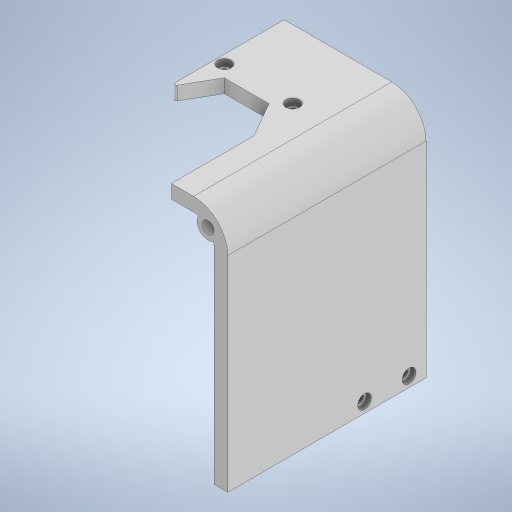
# Autodesk Inventor part: 배터리 커버
Saved by Autodesk Inventor 2023 (Build 270158000, 158)
## iProperties
Created: 2022-08-16
Part Number: 배터리 커버
Material: 일반
Document SubType Name: Modeling
Designer: fly01
Density: 1 g/cm^3
Appearance: 기본값
Author: fly01
Autodesk Inventor part; units mm, degrees
ref_plane "YZ Plane" through (0, 0, 0) normal (1, 0, 0) x (0, 1, 0)
ref_plane "XZ Plane" through (0, 0, 0) normal (0, 1, 0) x (-1, 0, 0)
ref_plane "XY Plane" through (0, 0, 0) normal (0, 0, 1) x (1, 0, 0)
sketch "스케치1" plane through (0, 0, 0) normal (0, 0, 1) x (1, 0, 0)
  line L0 (-7.2322, -10.1) -> (-7.2322, -70.1)
  line L1 (-17.2322, -0.1) -> (-48.7322, -0.1)
  line L2 (-34.3093, -4.1) -> (-17.2322, -4.1)
  line L3 (-11.2322, -10.1) -> (-11.2322, -70.1)
  line L4 (-48.7322, -0.1) -> (-48.7322, -4.1)
  line L5 (-48.7322, -4.1) -> (-34.3093, -4.1)
  line L6 (-11.2322, -70.1) -> (-7.2322, -70.1)
  arc A0 (-11.2322, -10.1) -> (-17.2322, -4.1) centre (-17.2322, -10.1) ccw
  arc A1 (-7.2322, -10.1) -> (-17.2322, -0.1) centre (-17.2322, -10.1) ccw
  point P0 (-7.2322, -0.1)
  dimension "d0" = 70
  dimension "d1" = 41.5
  dimension "d2" = 4
  dimension "d3" = 90
  dimension "d4" = 6
  dimension "d5" = 10
  constraints: 14 end point, 4 point on circle, 4 tangent, 3 horizontal, 2 centre point, 2 point on line, 1 vertical, 1 other
  measures "d0" distance of point (-7.232, -0.1) L0.end
  measures "d1" distance of point (-7.232, -0.1) L1.end
  measures "d2" distance between parallel lines of L1 L2
  measures "d3" angle of L4 L5
  measures "d4" radius of A0
  measures "d5" radius of A1
extrude "돌출1" add sketch "스케치1" along normal blind 23
sketch "스케치2" plane through (-7.2322, -70.1, 0) normal (1, 0, 0) x (0, 0, -1)
  line L0 (-23, 0) -> (-23, 60) projected
  line L1 (-23, 6) -> (0, 6)
  line L2 (0, 60) -> (0, 0) projected
  line L3 (0, 6) -> (0, 0)
  line L4 (0, 3) -> (-23, 3) construction
  line L5 (0, 0) -> (-23, 0) projected
  circle A0 centre (-18, 3) radius 1.25
  circle A1 centre (-5, 3) radius 1.25
  point P0 (0, 70.1)
  dimension "d8" = 6
  dimension "d9" = 2.5
  dimension "d10" = 2.5
  dimension "d11" = 5
  dimension "d12" = 5
  constraints: 6 end point, 4 point on line, 2 centre point, 2 perpendicular, 1 horizontal, 1 midpoint
  measures "d8" distance between parallel lines of L5 L1
  measures "d9" diameter of A0
  measures "d10" diameter of A1
  measures "d11" distance from line of L0 A0.centre
  measures "d12" distance from line of L2 A1.centre
extrude "돌출2" cut sketch "스케치2" against normal through all contours A0 | A1
sketch "스케치3" plane through (-7.2322, -70.1, 0) normal (1, 0, 0) x (0, 0, -1)
  circle A0 centre (-18, 3) radius 1.25 projected
  circle A1 centre (-18, 3) radius 2
  circle A2 centre (-5, 3) radius 1.25 projected
  circle A3 centre (-5, 3) radius 2
  point P0 (0, 70.1)
  dimension "d15" = 4
  dimension "d16" = 4
  constraints: 2 centre point, 2 coincident
  measures "d15" diameter of A1
  measures "d16" diameter of A3
extrude "돌출3" cut sketch "스케치3" against normal blind 1.5 contours A0 | A1 | A2 | A3
sketch "스케치4" plane through (-48.7322, -0.1, 0) normal (0, 1, 0) x (1, 0, 0)
  line L0 (0, -34.8253) -> (6.25, -24)
  line L1 (6.25, -24) -> (18.75, -24)
  line L2 (18.75, -24) -> (25, -34.8253)
  line L3 (25, -34.8253) -> (18.75, -45.6506)
  line L4 (18.75, -45.6506) -> (6.25, -45.6506)
  line L5 (6.25, -45.6506) -> (0, -34.8253)
  line L6 (0, 0) -> (0, -23) projected
  line L7 (0, -34.8253) -> (0, -23)
  line L8 (25, -34.8253) -> (25, -17.3222)
  line L9 (0, -23) -> (31.5, -23) projected
  line L10 (25.433, -34.5753) -> (19.0387, -23.5)
  line L11 (19.0387, -23.5) -> (5.9613, -23.5)
  line L12 (5.9613, -23.5) -> (-0.433, -34.5753)
  point P0 (48.7322, 0)
  point P1 (12.5, -34.8253)
  point P2 (15.75, -23)
  point P3 (25, -23)
  point P4 (25, -33.8253)
  point P5 (0, -33.8253)
  dimension "d19" = 25
  dimension "d20" = 1
  dimension "d23" = 0.5
  constraints: 22 end point, 2 vertical, 1 horizontal, 1 vertical alignment, 17 other
  measures "d19" distance of L2.end L0.start
  measures "d20" distance from line of point (15.75, -23) L1
  measures "d23" distance between parallel lines of L2 L10
extrude "돌출4" add sketch "스케치4" against normal blind 4 contours L7 L9 L8 L10 L11 L12
sketch "스케치5" plane through (0, 0, 23) normal (0, 0, 1) x (1, 0, 0)
  line L0 (-23.7322, -0.1) -> (-23.7322, -4.1) projected
  line L1 (-17.2322, -4.1) -> (-23.7322, -4.1) projected
  arc A0 (-11.2322, -10.1) -> (-17.2322, -4.1) centre (-17.2322, -10.1) ccw projected
  line L2 (-11.2322, -70.1) -> (-11.2322, -10.1) projected
  line L3 (-7.2322, -70.1) -> (-11.2322, -70.1) projected
  line L4 (-7.2322, -10.1) -> (-7.2322, -70.1) projected
  arc A1 (-7.2322, -10.1) -> (-17.2322, -0.1) centre (-17.2322, -10.1) ccw projected
  line L5 (-23.7322, -0.1) -> (-17.2322, -0.1) projected
  point P0 (0, 0)
extrude "돌출5" add sketch "스케치5" along normal blind 11
fillet "모깎기2" radius 0.5 1 edges at (-48.7322, -2.1, 33.8253)
sketch "스케치6" plane through (-48.7322, -0.1, 0) normal (0, 1, 0) x (1, 0, 0)
  circle A0 centre (2.5, -20) radius 1.25
  circle A1 centre (2.5, -20) radius 2
  line L0 (5.9613, -23.5) -> (19.0387, -23.5) projected
  line L1 (12.5, -23.5) -> (12.5, -5.5382)
  circle A2 centre (22.5, -20) radius 1.25
  circle A3 centre (22.5, -20) radius 2
  line L2 (31.5, 0) -> (0, 0) projected
  point P0 (48.7322, 0)
  dimension "d28" = 2.5
  dimension "d29" = 4
  dimension "d30" = 20
  dimension "d31" = 20
  constraints: 4 centre point, 2 coincident, 2 end point, 2 symmetric about line, 1 midpoint, 1 vertical, 2 other
  measures "d28" diameter of A0
  measures "d29" diameter of A1
  measures "d30" distance of A2.centre A0.centre
  measures "d31" distance from line of L2 A2.centre
extrude "돌출6" cut sketch "스케치6" against normal through all contours A0 | A2
extrude "돌출7" cut sketch "스케치6" against normal blind 2 contours A0 | A1 | A2 | A3
sketch "스케치7" plane through (0, 0, 34) normal (0, 0, 1) x (1, 0, 0)
  arc A0 (-7.2322, -10.1) -> (-17.2322, -0.1) centre (-17.2322, -10.1) ccw projected
  circle A1 centre (-12.9896, -5.8574) radius 3.25
  line L0 (-10.1611, -3.029) -> (-12.9896, -5.8574) construction
  arc A2 (-11.2322, -10.1) -> (-17.2322, -4.1) centre (-17.2322, -10.1) ccw construction
  line L1 (-11.2322, -70.1) -> (-11.2322, -10.1) projected
  circle A3 centre (-12.9896, -5.8574) radius 1.75
  point P0 (0, 0)
  dimension "d60" = 6.5
  dimension "d61" = 135
  dimension "d62" = 3.5
  constraints: 3 point on circle, 2 centre point, 2 coincident, 2 end point
  measures "d60" diameter of A1
  measures "d61" angle of L1 L0
  measures "d62" diameter of A3
extrude "돌출8" cut sketch "스케치7" against normal through all contours A3
extrude "돌출9" add sketch "스케치7" against normal blind 34
sketch "스케치8" plane through (-48.7322, -4.1, 0) normal (0, -1, 0) x (1, 0, 0)
  circle A0 centre (12.5, 9.5) radius 9.5
  line L0 (5.9613, 23.5) -> (19.0387, 23.5) projected
  line L1 (0, 0) -> (31.5, 0) projected
  point P0 (48.7322, 0)
  point P1 (12.5, 23.5)
  dimension "d42" = 19
  constraints: 1 centre point, 1 midpoint, 1 tangent, 1 vertical alignment
  measures "d42" diameter of A0
extrude "돌출10" cut sketch "스케치8" against normal blind 0.4
sketch "스케치9" plane through (0, 0, 34) normal (0, 0, 1) x (1, 0, 0)
  arc A0 (-11.2322, -10.1) -> (-11.3998, -8.692) centre (-17.2322, -10.1) ccw projected
  line L0 (-11.2322, -70.1) -> (-11.2322, -10.1) projected
  line L1 (-7.2322, -70.1) -> (-11.2322, -70.1) projected
  line L2 (-7.2322, -10.1) -> (-7.2322, -70.1) projected
  arc A1 (-7.2322, -10.1) -> (-17.2322, -0.1) centre (-17.2322, -10.1) ccw projected
  line L3 (-23.7322, -0.1) -> (-17.2322, -0.1) projected
  line L4 (-23.7322, -4.1) -> (-23.7322, -0.1) projected
  line L5 (-17.2322, -4.1) -> (-23.7322, -4.1) projected
  circle A2 centre (-12.9896, -5.8574) radius 1.75 projected
  arc A3 (-15.8242, -4.2676) -> (-17.2322, -4.1) centre (-17.2322, -10.1) ccw projected
  arc A4 (-15.8242, -4.2676) -> (-11.3998, -8.692) centre (-12.9896, -5.8574) ccw projected
  point P0 (0, 0)
extrude "돌출11" add sketch "스케치9" along normal blind 24
